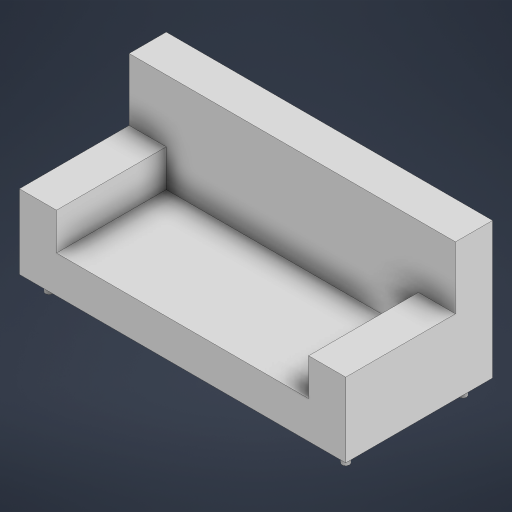
# Autodesk Inventor part: Divano Valdinoce
Saved by Autodesk Inventor 2024.2 (Build 282272000, 272)
## iProperties
Created: 2025-08-18
Part Number: Divano Valdinoce
Material: Generic
Document SubType Name: Modeling
Designer: Luca
Density: 1 g/cm^3
Appearance: Default
Author: Luca
Autodesk Inventor part; units mm, degrees
ref_plane "YZ Plane" through (0, 0, 0) normal (1, 0, 0) x (0, 1, 0)
ref_plane "XZ Plane" through (0, 0, 0) normal (0, 1, 0) x (-1, 0, 0)
ref_plane "XY Plane" through (0, 0, 0) normal (0, 0, 1) x (1, 0, 0)
sketch "Sketch1" plane through (0, 0, 0) normal (0, 1, 0) x (-1, 0, 0)
  line L0 (1100, 990) -> (-1100, 990)
  line L1 (-1100, 990) -> (-1100, 0)
  line L2 (-1100, 0) -> (1100, 0)
  line L3 (1100, 0) -> (1100, 990)
  point P0 (0, 0)
  point P1 (0, 0)
  dimension "d0" = 2200
  dimension "d1" = 990
  constraints: 8 end point, 2 parallel, 1 coincident, 1 horizontal, 1 midpoint, 1 perpendicular
  measures "d0" distance of L2.end L1.end
  measures "d1" distance of L1.end L0.end
extrude "Extrusion1" add sketch "Sketch1" along normal blind 1020
sketch "Sketch2" plane through (1100, 0, 990) normal (1, 0, 0) x (0, 0, -1)
  line L0 (0, 0) -> (0, 1020) projected
  line L1 (0, 1020) -> (740, 1020)
  line L2 (740, 1020) -> (740, 600)
  line L3 (740, 600) -> (0, 600)
  line L4 (0, 600) -> (0, 1020)
  line L5 (990, 0) -> (990, 1020) projected
  point P0 (0, 600)
  dimension "d4" = 600
  dimension "d5" = 250
  constraints: 8 end point, 2 parallel, 1 horizontal, 1 perpendicular
  measures "d4" distance from line of L0.start L3
  measures "d5" distance between parallel lines of L5 L2
extrude "Extrusion2" cut sketch "Sketch2" against normal through all
sketch "Sketch3" plane through (1100, 600, 990) normal (0, 1, 0) x (1, 0, 0)
  line L0 (-2200, 0) -> (0, 0) projected
  line L1 (-2200, 740) -> (0, 740) projected
  line L2 (-1950, 0) -> (-250, 0)
  line L3 (-250, 0) -> (-250, 740)
  line L4 (-250, 740) -> (-1950, 740)
  line L5 (-1950, 740) -> (-1950, 0)
  line L6 (-2200, 0) -> (-2200, 740) projected
  point P0 (-1100, 990)
  point P1 (-1100, 0)
  point P2 (-1100, 0)
  point P3 (-1950, 740)
  point P4 (-250, 0)
  dimension "d8" = 250
  constraints: 8 end point, 2 midpoint, 2 parallel, 2 point on line, 1 coincident, 1 horizontal, 1 perpendicular
  measures "d8" distance between parallel lines of L6 L5
extrude "Extrusion3" cut sketch "Sketch3" against normal blind 250 contours L5 L1 L3 L0
sketch "Sketch4" plane through (0, 0, 0) normal (0, -1, 0) x (1, 0, 0)
  line L0 (1100, 990) -> (1100, 0) projected
  line L1 (-1100, 990) -> (1100, 990) projected
  line L2 (-1100, 0) -> (-1100, 990) projected
  line L3 (1100, 0) -> (-1100, 0) projected
  line L4 (1000, 890) -> (1000, 100) construction
  line L5 (1000, 100) -> (-1000, 100) construction
  line L6 (-1000, 100) -> (-1000, 890) construction
  line L7 (-1000, 890) -> (1000, 890) construction
  circle A0 centre (-1000, 890) radius 25
  circle A1 centre (1000, 890) radius 25
  circle A2 centre (1000, 100) radius 25
  circle A3 centre (-1000, 100) radius 25
  point P0 (0, 0)
  dimension "d11" = 100
  dimension "d12" = 50
  dimension "d13" = 50
  dimension "d14" = 50
  dimension "d15" = 50
  constraints: 8 end point, 4 centre point, 4 coincident, 3 other
  measures "d11" distance between parallel lines of L1 L7
  measures "d12" diameter of A0
  measures "d13" diameter of A1
  measures "d14" diameter of A2
  measures "d15" diameter of A3
extrude "Extrusion4" cut sketch "Sketch4" against normal blind 100
body "Solid1"
